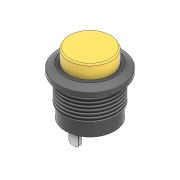
# Autodesk Inventor part: knop op en neer
Saved by Autodesk Inventor 2020.3 (Build 243373000, 373)
## iProperties
Created: 2020-12-08
Part Number: knop op en neer
Material: ABS Plastic
Document SubType Name: Modeling
Designer: Svend
Density: 1.06 g/cm^3
Appearance: Smooth - White
Author: Svend
Autodesk Inventor part; units mm, degrees
ref_plane "YZ Plane" through (0, 0, 0) normal (1, 0, 0) x (0, 1, 0)
ref_plane "XZ Plane" through (0, 0, 0) normal (0, 1, 0) x (-1, 0, 0)
ref_plane "XY Plane" through (0, 0, 0) normal (0, 0, 1) x (1, 0, 0)
sketch "Sketch1" plane through (0, 0, 0) normal (0, 0, 1) x (1, 0, 0)
  arc A0 (6.5, 18.5) -> (0, 19.5) centre (0, -2.125) ccw
  line L0 (0, 19.5) -> (0, 0)
  line L1 (6.5, 18.5) -> (6.5, 14.5)
  line L2 (6.5, 14.5) -> (7.5, 14.5)
  line L3 (7.5, 14.5) -> (9.6, 13.2876)
  line L4 (9.6, 13.2876) -> (9.6, 11.7876)
  line L5 (9.6, 11.7876) -> (8, 11.7876)
  line L6 (8, 11.7876) -> (8, 4.2813)
  line L7 (8, 4.2813) -> (7.5, 4.2813)
  line L8 (7.5, 4.2813) -> (7.5, 0)
  line L9 (7.5, 0) -> (0, 0)
  dimension "d0" = 19.5
  dimension "d1" = 18.5
  dimension "d2" = 6.5
  dimension "d3" = 4
  dimension "d4" = 1
  dimension "d5" = 30
  dimension "d6" = 9.6
  dimension "d7" = 1.5
  dimension "d8" = 8
  dimension "d9" = 7.5
  constraints: 20 end point, 5 perpendicular, 4 vertical, 2 point on circle, 1 centre point, 1 line through centre
  measures "d0" distance of L0.start L0.end
  measures "d1" vertical distance of L0.end L1.start
  measures "d2" distance from line of L0 L1.start
  measures "d3" distance of L1.start L1.end
  measures "d4" distance of L1.end L2.end
  measures "d5" angle of L2 L3
  measures "d6" distance from line of L0 L3.end
  measures "d7" distance of L3.end L4.end
  measures "d8" distance from line of L0 L5.end
  measures "d9" distance between parallel lines of L0 L8
revolve "Revolution1" add sketch "Sketch1" angle 360 about axis through (0, 19.5, 0) along (0, -1, 0)
thread "Thread1" size "M16x1" class "6g" standard "ISO Metric profile" full length
sketch "Sketch2" plane through (0, 0, 0) normal (0, -1, 0) x (1, 0, 0)
  circle A0 centre (0, 0) radius 7.5 projected
  line L0 (1.5, 5) -> (-1.5, 5)
  line L1 (-1.5, 5) -> (-1.5, 4)
  line L2 (-1.5, 4) -> (1.5, 4)
  line L3 (1.5, 4) -> (1.5, 5)
  circle A1 centre (0, 0) radius 7.5 construction
  line L4 (7.5, 0) -> (-7.5, 0) construction
  line L5 (1.5, -5) -> (-1.5, -5)
  line L6 (-1.5, -5) -> (-1.5, -4)
  line L7 (-1.5, -4) -> (1.5, -4)
  line L8 (1.5, -4) -> (1.5, -5)
  point P0 (0, 0)
  point P1 (0, 4)
  point P2 (0, -4)
  dimension "d13" = 3
  dimension "d14" = 1
  dimension "d15" = 4
  constraints: 18 end point, 5 symmetric about line, 2 horizontal, 2 midpoint, 2 parallel, 2 point on circle, 1 coincident, 1 perpendicular, 1 vertical alignment
  measures "d13" distance of L0.start L0.end
  measures "d14" distance of L2.end L0.start
  measures "d15" distance from line of point (0, 0) L2
extrude "Extrusion1" add sketch "Sketch2" along normal blind 5 contours L3 L2 L1 L0 | L5 L6 L7 L8
fillet "Fillet1" radius 1 4 edges at (1.5, -5, 4.5) (-1.5, -5, 4.5) (1.5, -5, -4.5) (-1.5, -5, -4.5)
fillet "Fillet2" radius 0.2 7 edges at (-7.5, 0, 0) (-7.5, 14.5, 0) (-9.6, 13.2876, 0) (-9.6, 11.7876, 0) (-8, 11.7876, 0) (-8, 4.2813, 0) (-7.5, 4.2813, 0)
fillet "Fillet3" radius 0.5 1 edges at (-6.5, 18.5, 0)
fillet "Fillet4" radius 0.1 20 edges at (1.2071, -4.7071, -5) (0, -5, -5) (-1.2071, -4.7071, -5) (-1.5, -2, -5) (1.5, -2, -5) (0, -5, -4) (-1.2071, -4.7071, -4) (-1.5, -2, -4) (1.5, -2, -4) (1.2071, -4.7071, -4) (-1.2071, -4.7071, 4) (0, -5, 4) (1.2071, -4.7071, 4) (1.5, -2, 4) (-1.5, -2, 4) (0, -5, 5) (-1.2071, -4.7071, 5) (-1.5, -2, 5) (1.5, -2, 5) (1.2071, -4.7071, 5)
body "Solid1"
